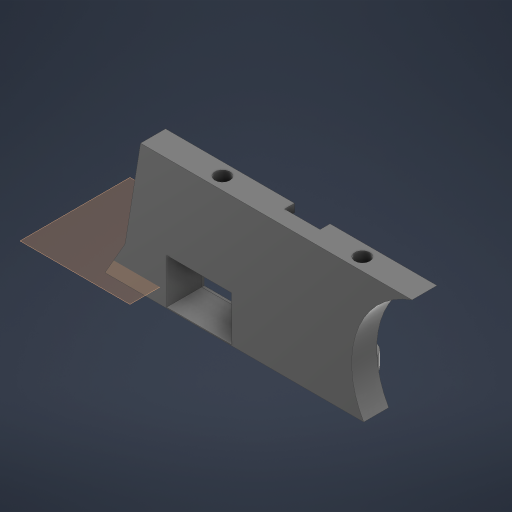
# Autodesk Inventor part: bok_lewy
Saved by Autodesk Inventor 2024 (Build 280153000, 153)
## iProperties
Created: 2024-05-25
Part Number: bok_lewy
Material: ABS Plastic
Document SubType Name: Modeling
Designer: Adam
Density: 1.06 g/cm^3
Appearance: Smooth - White
Mass: 4.70038 g
Surface Area: 30.9781 cm^2
Volume: 4.70038 cm^3
Author: Adam
Autodesk Inventor part; units mm, degrees
ref_plane "YZ Plane" through (0, 0, 0) normal (1, 0, 0) x (0, 1, 0)
ref_plane "XZ Plane" through (0, 0, 0) normal (0, 1, 0) x (-1, 0, 0)
ref_plane "XY Plane" through (0, 0, 0) normal (0, 0, 1) x (1, 0, 0)
sketch "Sketch1" plane through (0, 0, 0) normal (0, 0, 1) x (1, 0, 0)
  line L0 (61.4575, 26) -> (7.1245, 26)
  line L1 (7.1245, 26) -> (4.1002, 7.362)
  line L2 (51.7851, 0) -> (0, 0)
  line L3 (0, 0) -> (3.8581, 6.6824)
  arc A0 (61.4575, 26) -> (51.7851, 0) centre (67.3735, 9) ccw
  arc A1 (3.8581, 6.6824) -> (4.1002, 7.362) centre (2.126, 7.6824) ccw
  constraints: 8 end point, 4 point on circle, 2 centre point, 1 horizontal
extrude "Extrusion1" add sketch "Sketch1" along normal blind 5
ref_plane "Work Plane1" through (0, 3, 0) normal (0, 1, 0) x (1, 0, 0)
sketch "Sketch4" plane through (0, 0, 5) normal (0, 0, 1) x (1, 0, 0)
  line L0 (14.8454, 6.6801) -> (22.8454, 6.6801)
  line L1 (22.8454, 6.6801) -> (22.8454, 2.6801)
  line L2 (22.8454, 2.6801) -> (14.8454, 2.6801)
  line L3 (14.8454, 2.6801) -> (14.8454, 6.6801)
  line L4 (14.8454, 6.6801) -> (22.8454, 2.6801) construction
  line L5 (22.8454, 6.6801) -> (14.8454, 2.6801) construction
  point P0 (0, 0)
  point P1 (18.8454, 4.6801)
  dimension "d31" = 8
  dimension "d32" = 4
  constraints: 12 end point, 2 midpoint, 2 parallel, 1 horizontal, 1 perpendicular
  measures "d31" distance of L1.end L2.end
  measures "d32" distance of L0.end L1.end
extrude "Extrusion4" cut sketch "Sketch4" against normal blind 5
chamfer "Chamfer2" distance 2.5 distance2 4.5 4 edges at (18.8454, 6.6801, 5) (14.8454, 4.6801, 5) (18.8454, 2.6801, 5) (22.8454, 4.6801, 5) measured on face at (18.8454, 2.1801, 5) measured on face at (18.8454, 7.1801, 5) measured on face at (14.3454, 4.6801, 5) measured on face at (23.3454, 4.6801, 5)
sketch "Sketch6" plane through (0, 0, 0) normal (0, 0, -1) x (-1, 0, 0)
  line L0 (-30.1514, 18.0264) -> (-42.8514, 18.0264)
  line L1 (-42.8514, 24.3764) -> (-30.1514, 24.3764)
  line L2 (-32.9514, 24.3764) -> (-32.9514, 30.7164)
  line L3 (-40.0514, 24.3764) -> (-40.0514, 30.7164)
  line L4 (-40.0514, 30.7164) -> (-32.9514, 30.7164)
  line L5 (-42.8514, 24.3764) -> (-42.8514, 18.0264)
  line L6 (-30.1514, 24.3764) -> (-30.1514, 18.0264)
  point P0 (0, 0)
  dimension "d39" = 12.7
  dimension "d41" = 12.7
  dimension "d42" = 6.35
  constraints: 14 end point, 2 perpendicular, 2 vertical
  measures "d39" distance of L1.start L1.end
  measures "d41" distance of L0.end L0.start
  measures "d42" distance of L1.start L0.end
extrude "Extrusion5" cut sketch "Sketch6" against normal blind 2
sketch "Sketch7" plane through (0, 0, 2) normal (0, 0, -1) x (-1, 0, 0)
  line L0 (-42.8514, 18.0264) -> (-42.8514, 24.3764) projected
  line L1 (-30.1514, 24.3764) -> (-30.1514, 18.0264) projected
  line L2 (-42.8514, 24.3764) -> (-30.1514, 24.3764)
  line L3 (-30.1514, 24.3764) -> (-30.1514, 18.0264)
  line L4 (-30.1514, 18.0264) -> (-42.8514, 18.0264)
  line L5 (-42.8514, 18.0264) -> (-42.8514, 24.3764)
  point P0 (0, 0)
  constraints: 8 end point, 2 parallel, 1 horizontal, 1 perpendicular
extrude "Extrusion6" cut sketch "Sketch7" against normal blind 1.3
chamfer "Chamfer3" distance 8 angle 20 1 edges at (36.5014, 18.0264, 0) measured on face at (36.5014, 17.5264, 0)
sketch "Sketch9" plane through (0, 0, 0) normal (0, -1, 0) x (1, 0, 0)
  line L0 (44.7851, -7) -> (44.7851, 0) projected
  line L1 (36.7851, -7) -> (44.7851, -7) projected
  circle A0 centre (40.7851, -3) radius 1.55 projected
  circle A1 centre (40.7851, -3) radius 1.55
  line L2 (44.7851, 0) -> (36.7851, 0)
  line L3 (36.7851, 0) -> (36.7851, -7)
  line L4 (36.7851, -7) -> (44.7851, -7)
  line L5 (44.7851, -7) -> (44.7851, 0)
  point P0 (0, 0)
  constraints: 8 end point, 2 parallel, 1 centre point, 1 coincident, 1 concentric, 1 horizontal, 1 perpendicular
extrude "Extrusion8" add sketch "Sketch9" against normal blind 3
sketch "Sketch10" plane through (7.1245, 26, 5) normal (0, 1, 0) x (1, 0, 0)
  circle A0 centre (13.8867, 2.5) radius 1.5 projected
  circle A1 centre (41.8867, 2.5) radius 1.5 projected
  circle A2 centre (13.8867, 2.5) radius 1.5
  circle A3 centre (41.8867, 2.5) radius 1.5
  point P0 (-7.1245, 5)
  constraints: 2 centre point, 2 coincident, 2 concentric
extrude "Extrusion9" cut sketch "Sketch10" against normal blind 2
sketch "Sketch11" plane through (0, 3, 0) normal (0, 1, 0) x (1, 0, 0)
  line L0 (37.7801, 3) -> (39.2826, 5.6024) projected
  line L1 (39.2826, 0.3976) -> (37.7801, 3) projected
  line L2 (37.7801, 3) -> (39.2826, 5.6024)
  line L3 (39.2826, 5.6024) -> (42.2876, 5.6024)
  line L4 (42.2876, 5.6024) -> (43.7901, 3)
  line L5 (43.7901, 3) -> (42.2876, 0.3976)
  line L6 (42.2876, 0.3976) -> (39.2826, 0.3976)
  line L7 (39.2826, 0.3976) -> (37.7801, 3)
  circle A0 centre (40.7851, 3) radius 1.55
  point P0 (0, 0)
  constraints: 12 end point, 2 coincident, 1 centre point, 13 other
extrude "Extrusion10" cut sketch "Sketch11" against normal blind 2
fillet "Fillet3" radius 3 5 edges at (40.7851, 3, 0) (36.7851, 1.5, 0) (44.7851, 1.5, 0) (44.7851, 1.5, -7) (36.7851, 1.5, -7)
body "Solid1"
